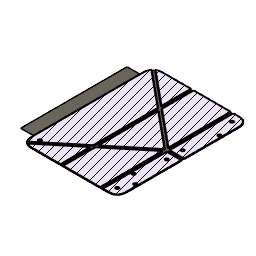
Ipad Case v1 (Autodesk Fusion 360 archive; units mm, degrees)
design "Ipad Cover v2"
part number: 2026-04-06-16-04-37-224
Autodesk Fusion 360 part; units mm, degrees
note: some values were not read from the file. Chosen so that the rebuilt part matches the saved one: which bodies a step acts on. Set by a fixed rule: which sketch regions a step uses.
sketch "Sketch1" plane through (0, 0, 0) normal (0, 0, 1) x (1, 0, 0)
  line L0 (22.75, 0) -> (156.76, 0)
  line L1 (179.51, 22.75) -> (179.51, 223.88)
  line L2 (156.76, 246.63) -> (22.75, 246.63)
  line L3 (0, 223.8801) -> (0, 22.75)
  spline S0 degree 5 poles (22.75, 0) (16.7, 0.14) (14.9, 0.32) (11.36, 0.69) (10.05, 1.08) (8.75, 1.6) (7.46, 2.26) (6.23, 3.06) (5.07, 4) (4.01, 5.05) (3.08, 6.21) (2.27, 7.44) (1.61, 8.73) (1, 10.3) (0.58, 11.86) (0.3, 13.37) (0.14, 14.82) (0.06, 16.18) (0, 22.75) knots 0 0 0 0 0 0 0.071429 0.142857 0.214286 0.285714 0.357143 0.428571 0.5 0.571429 0.642857 0.714286 0.785714 0.857143 0.928571 1 1 1 1 1 1
  line L4 (22.75, 0) -> (16.7, 0.14) construction
  line L5 (16.7, 0.14) -> (14.9, 0.32) construction
  line L6 (14.9, 0.32) -> (11.36, 0.69) construction
  line L7 (11.36, 0.69) -> (10.05, 1.08) construction
  line L8 (10.05, 1.08) -> (8.75, 1.6) construction
  line L9 (8.75, 1.6) -> (7.46, 2.26) construction
  line L10 (7.46, 2.26) -> (6.23, 3.06) construction
  line L11 (6.23, 3.06) -> (5.07, 4) construction
  line L12 (5.07, 4) -> (4.01, 5.05) construction
  line L13 (4.01, 5.05) -> (3.08, 6.21) construction
  line L14 (3.08, 6.21) -> (2.27, 7.44) construction
  line L15 (2.27, 7.44) -> (1.61, 8.73) construction
  line L16 (1.61, 8.73) -> (1, 10.3) construction
  line L17 (1, 10.3) -> (0.58, 11.86) construction
  line L18 (0.58, 11.86) -> (0.3, 13.37) construction
  line L19 (0.3, 13.37) -> (0.14, 14.82) construction
  line L20 (0.14, 14.82) -> (0.06, 16.18) construction
  line L21 (0.06, 16.18) -> (0, 22.75) construction
  spline S1 degree 5 poles (22.75, 0) (16.7, 0.14) (14.9, 0.32) (11.36, 0.69) (10.05, 1.08) (8.75, 1.6) (7.46, 2.26) (6.23, 3.06) (5.07, 4) (4.01, 5.05) (3.08, 6.21) (2.27, 7.44) (1.61, 8.73) (1, 10.3) (0.58, 11.86) (0.3, 13.37) (0.14, 14.82) (0.06, 16.18) (0, 22.75) knots 0 0 0 0 0 0 0.071429 0.142857 0.214286 0.285714 0.357143 0.428571 0.5 0.571429 0.642857 0.714286 0.785714 0.857143 0.928571 1 1 1 1 1 1
  line L22 (22.75, 0) -> (16.7, 0.14) construction
  line L23 (16.7, 0.14) -> (14.9, 0.32) construction
  line L24 (14.9, 0.32) -> (11.36, 0.69) construction
  line L25 (11.36, 0.69) -> (10.05, 1.08) construction
  line L26 (10.05, 1.08) -> (8.75, 1.6) construction
  line L27 (8.75, 1.6) -> (7.46, 2.26) construction
  line L28 (7.46, 2.26) -> (6.23, 3.06) construction
  line L29 (6.23, 3.06) -> (5.07, 4) construction
  line L30 (5.07, 4) -> (4.01, 5.05) construction
  line L31 (4.01, 5.05) -> (3.08, 6.21) construction
  line L32 (3.08, 6.21) -> (2.27, 7.44) construction
  line L33 (2.27, 7.44) -> (1.61, 8.73) construction
  line L34 (1.61, 8.73) -> (1, 10.3) construction
  line L35 (1, 10.3) -> (0.58, 11.86) construction
  line L36 (0.58, 11.86) -> (0.3, 13.37) construction
  line L37 (0.3, 13.37) -> (0.14, 14.82) construction
  line L38 (0.14, 14.82) -> (0.06, 16.18) construction
  line L39 (0.06, 16.18) -> (0, 22.75) construction
  spline S2 degree 5 poles (0, 223.88) (0, 223.8801) (0, 223.8802) (0, 223.8803) (0, 223.8804) (0, 223.8804) knots 0 0 0 0 0 0 0.000083 0.000083 0.000083 0.000083 0.000083 0.000083
  line L40 (0, 223.88) -> (0, 223.88)
  line L41 (0, 223.8804) -> (0, 223.8805)
  line L42 (89.755, 246.63) -> (89.755, 0) construction
  line L43 (179.51, 123.315) -> (0, 123.315) construction
  spline S3 degree 5 poles (156.76, 0) (162.81, 0.14) (164.61, 0.32) (168.15, 0.69) (169.46, 1.08) (170.76, 1.6) (172.05, 2.26) (173.28, 3.06) (174.44, 4) (175.5, 5.05) (176.43, 6.21) (177.24, 7.44) (177.9, 8.73) (178.51, 10.3) (178.93, 11.86) (179.21, 13.37) (179.37, 14.82) (179.45, 16.18) (179.51, 22.75) knots 0 0 0 0 0 0 0.071429 0.142857 0.214286 0.285714 0.357143 0.428571 0.5 0.571429 0.642857 0.714286 0.785714 0.857143 0.928571 1 1 1 1 1 1
  line L44 (156.76, 0) -> (162.81, 0.14) construction
  line L45 (162.81, 0.14) -> (164.61, 0.32) construction
  line L46 (164.61, 0.32) -> (168.15, 0.69) construction
  line L47 (168.15, 0.69) -> (169.46, 1.08) construction
  line L48 (169.46, 1.08) -> (170.76, 1.6) construction
  line L49 (170.76, 1.6) -> (172.05, 2.26) construction
  line L50 (172.05, 2.26) -> (173.28, 3.06) construction
  line L51 (173.28, 3.06) -> (174.44, 4) construction
  line L52 (174.44, 4) -> (175.5, 5.05) construction
  line L53 (175.5, 5.05) -> (176.43, 6.21) construction
  line L54 (176.43, 6.21) -> (177.24, 7.44) construction
  line L55 (177.24, 7.44) -> (177.9, 8.73) construction
  line L56 (177.9, 8.73) -> (178.51, 10.3) construction
  line L57 (178.51, 10.3) -> (178.93, 11.86) construction
  line L58 (178.93, 11.86) -> (179.21, 13.37) construction
  line L59 (179.21, 13.37) -> (179.37, 14.82) construction
  line L60 (179.37, 14.82) -> (179.45, 16.18) construction
  line L61 (179.45, 16.18) -> (179.51, 22.75) construction
  spline S4 degree 5 poles (156.76, 246.63) (162.81, 246.49) (164.61, 246.31) (168.15, 245.94) (169.46, 245.55) (170.76, 245.03) (172.05, 244.37) (173.28, 243.57) (174.44, 242.63) (175.5, 241.58) (176.43, 240.42) (177.24, 239.19) (177.9, 237.9) (178.51, 236.33) (178.93, 234.77) (179.21, 233.26) (179.37, 231.81) (179.45, 230.45) (179.51, 223.88) knots 0 0 0 0 0 0 0.071429 0.142857 0.214286 0.285714 0.357143 0.428571 0.5 0.571429 0.642857 0.714286 0.785714 0.857143 0.928571 1 1 1 1 1 1
  line L62 (156.76, 246.63) -> (162.81, 246.49) construction
  line L63 (162.81, 246.49) -> (164.61, 246.31) construction
  line L64 (164.61, 246.31) -> (168.15, 245.94) construction
  line L65 (168.15, 245.94) -> (169.46, 245.55) construction
  line L66 (169.46, 245.55) -> (170.76, 245.03) construction
  line L67 (170.76, 245.03) -> (172.05, 244.37) construction
  line L68 (172.05, 244.37) -> (173.28, 243.57) construction
  line L69 (173.28, 243.57) -> (174.44, 242.63) construction
  line L70 (174.44, 242.63) -> (175.5, 241.58) construction
  line L71 (175.5, 241.58) -> (176.43, 240.42) construction
  line L72 (176.43, 240.42) -> (177.24, 239.19) construction
  line L73 (177.24, 239.19) -> (177.9, 237.9) construction
  line L74 (177.9, 237.9) -> (178.51, 236.33) construction
  line L75 (178.51, 236.33) -> (178.93, 234.77) construction
  line L76 (178.93, 234.77) -> (179.21, 233.26) construction
  line L77 (179.21, 233.26) -> (179.37, 231.81) construction
  line L78 (179.37, 231.81) -> (179.45, 230.45) construction
  line L79 (179.45, 230.45) -> (179.51, 223.88) construction
  spline S5 degree 5 poles (22.75, 246.63) (16.7, 246.49) (14.9, 246.31) (11.36, 245.94) (10.05, 245.55) (8.75, 245.03) (7.46, 244.37) (6.23, 243.57) (5.07, 242.63) (4.01, 241.58) (3.08, 240.42) (2.27, 239.19) (1.61, 237.9) (1, 236.33) (0.58, 234.77) (0.3, 233.26) (0.14, 231.81) (0.06, 230.45) (0, 223.88) knots 0 0 0 0 0 0 0.071429 0.142857 0.214286 0.285714 0.357143 0.428571 0.5 0.571429 0.642857 0.714286 0.785714 0.857143 0.928571 1 1 1 1 1 1
  line L80 (22.75, 246.63) -> (16.7, 246.49) construction
  line L81 (16.7, 246.49) -> (14.9, 246.31) construction
  line L82 (14.9, 246.31) -> (11.36, 245.94) construction
  line L83 (11.36, 245.94) -> (10.05, 245.55) construction
  line L84 (10.05, 245.55) -> (8.75, 245.03) construction
  line L85 (8.75, 245.03) -> (7.46, 244.37) construction
  line L86 (7.46, 244.37) -> (6.23, 243.57) construction
  line L87 (6.23, 243.57) -> (5.07, 242.63) construction
  line L88 (5.07, 242.63) -> (4.01, 241.58) construction
  line L89 (4.01, 241.58) -> (3.08, 240.42) construction
  line L90 (3.08, 240.42) -> (2.27, 239.19) construction
  line L91 (2.27, 239.19) -> (1.61, 237.9) construction
  line L92 (1.61, 237.9) -> (1, 236.33) construction
  line L93 (1, 236.33) -> (0.58, 234.77) construction
  line L94 (0.58, 234.77) -> (0.3, 233.26) construction
  line L95 (0.3, 233.26) -> (0.14, 231.81) construction
  line L96 (0.14, 231.81) -> (0.06, 230.45) construction
  line L97 (0.06, 230.45) -> (0, 223.88) construction
  dimension "d13" = 22.75
  dimension "d14" = 16.7
  dimension "d15" = 14.9
  dimension "d16" = 11.36
  dimension "d17" = 10.05
  dimension "d18" = 8.75
  dimension "d19" = 7.46
  dimension "d20" = 6.23
  dimension "d21" = 5.07
  dimension "d22" = 4.01
  dimension "d23" = 3.08
  dimension "d24" = 2.27
  dimension "d25" = 1.61
  dimension "d26" = 1
  dimension "d27" = 0.58
  dimension "d28" = 0.3
  dimension "d29" = 0.14
  dimension "d30" = 0.06
  dimension "d31" = 0.14
  dimension "d32" = 0.32
  dimension "d33" = 0.69
  dimension "d34" = 1.08
  dimension "d35" = 1.6
  dimension "d36" = 2.26
  dimension "d37" = 3.06
  dimension "d38" = 4
  dimension "d39" = 5.05
  dimension "d40" = 6.21
  dimension "d41" = 7.44
  dimension "d42" = 8.73
  dimension "d43" = 10.3
  dimension "d44" = 11.86
  dimension "d45" = 13.37
  dimension "d46" = 14.82
  dimension "d47" = 16.18
  dimension "d48" = 22.75
  constraint horizontal L0
  constraint vertical L1
  constraint horizontal L2
  constraint vertical L3
  constraint coincident L3 S2.start
  constraint coincident L3 S2.end
  constraint midpoint S2.start L40
  constraint midpoint S2.end L41
  constraint symmetric L0.start L42 L0.end
  constraint symmetric L3.end L42 L1.start
  constraint symmetric S1 L42 S3
  constraint symmetric L0.start L43 L2.end
  constraint symmetric L3.end L43 S2.start
  constraint symmetric S0 L43 S5
  constraint symmetric L43 L0.end L2.start
  constraint symmetric L43 L1.start L1.end
  constraint symmetric L43 S3 S4
  constraint coincident S2 L3.start
  measures "d13" distance of L3 L0.start
  measures "d14" distance of L3 L4.end
  measures "d15" distance of L3 L5.end
  measures "d16" distance of L3 L6.end
  measures "d17" distance of L3 L7.end
  measures "d18" distance of L3 L8.end
  measures "d19" distance of L3 L9.end
  measures "d20" distance of L3 L10.end
  measures "d21" distance of L3 L11.end
  measures "d22" distance of L3 L12.end
  measures "d23" distance of L3 L13.end
  measures "d24" distance of L3 L14.end
  measures "d25" distance of L3 L15.end
  measures "d26" distance of L3 L16.end
  measures "d27" distance of L3 L17.end
  measures "d28" distance of L3 L18.end
  measures "d29" distance of L3 L19.end
  measures "d30" distance of L3 L20.end
  measures "d31" distance of L0 L4.end
  measures "d32" distance of L0 L5.end
  measures "d33" distance of L0 L6.end
  measures "d34" distance of L0 L7.end
  measures "d35" distance of L0 L8.end
  measures "d36" distance of L0 L9.end
  measures "d37" distance of L0 L10.end
  measures "d38" distance of L0 L11.end
  measures "d39" distance of L0 L12.end
  measures "d40" distance of L0 L13.end
  measures "d41" distance of L0 L14.end
  measures "d42" distance of L0 L15.end
  measures "d43" distance of L0 L16.end
  measures "d44" distance of L0 L17.end
  measures "d45" distance of L0 L18.end
  measures "d46" distance of L0 L19.end
  measures "d47" distance of L0 L20.end
  measures "d48" distance of L0 L3.end
sketch "Sketch2" plane through (0, 0, 0) normal (0, 0, 1) x (1, 0, 0)
  line L0 (22.75, 0) -> (156.76, 0)
  line L1 (179.51, 22.75) -> (179.51, 223.88)
  spline S0 degree 5 poles (156.76, 0) (162.81, 0.14) (164.61, 0.32) (168.15, 0.69) (169.46, 1.08) (170.76, 1.6) (172.05, 2.26) (173.28, 3.06) (174.44, 4) (175.5, 5.05) (176.43, 6.21) (177.24, 7.44) (177.9, 8.73) (178.51, 10.3) (178.93, 11.86) (179.21, 13.37) (179.37, 14.82) (179.45, 16.18) (179.51, 22.75) knots 0 0 0 0 0 0 0.071429 0.142857 0.214286 0.285714 0.357143 0.428571 0.5 0.571429 0.642857 0.714286 0.785714 0.857143 0.928571 1 1 1 1 1 1
  spline S1 degree 5 poles (22.75, 0) (16.7, 0.14) (14.9, 0.32) (11.36, 0.69) (10.05, 1.08) (8.75, 1.6) (7.46, 2.26) (6.23, 3.06) (5.07, 4) (4.01, 5.05) (3.08, 6.21) (2.27, 7.44) (1.61, 8.73) (1, 10.3) (0.58, 11.86) (0.3, 13.37) (0.14, 14.82) (0.06, 16.18) (0, 22.75) knots 0 0 0 0 0 0 0.071429 0.142857 0.214286 0.285714 0.357143 0.428571 0.5 0.571429 0.642857 0.714286 0.785714 0.857143 0.928571 1 1 1 1 1 1
  line L2 (0, 223.8801) -> (0, 22.75)
  line L3 (156.76, 246.63) -> (22.75, 246.63)
  spline S2 degree 5 poles (156.76, 246.63) (162.81, 246.49) (164.61, 246.31) (168.15, 245.94) (169.46, 245.55) (170.76, 245.03) (172.05, 244.37) (173.28, 243.57) (174.44, 242.63) (175.5, 241.58) (176.43, 240.42) (177.24, 239.19) (177.9, 237.9) (178.51, 236.33) (178.93, 234.77) (179.21, 233.26) (179.37, 231.81) (179.45, 230.45) (179.51, 223.88) knots 0 0 0 0 0 0 0.071429 0.142857 0.214286 0.285714 0.357143 0.428571 0.5 0.571429 0.642857 0.714286 0.785714 0.857143 0.928571 1 1 1 1 1 1
  spline S3 degree 5 poles (22.75, 246.63) (16.7, 246.49) (14.9, 246.31) (11.36, 245.94) (10.05, 245.55) (8.75, 245.03) (7.46, 244.37) (6.23, 243.57) (5.07, 242.63) (4.01, 241.58) (3.08, 240.42) (2.27, 239.19) (1.61, 237.9) (1, 236.33) (0.58, 234.77) (0.3, 233.26) (0.14, 231.81) (0.06, 230.45) (0, 223.88) knots 0 0 0 0 0 0 0.071429 0.142857 0.214286 0.285714 0.357143 0.428571 0.5 0.571429 0.642857 0.714286 0.785714 0.857143 0.928571 1 1 1 1 1 1
  line L4 (22.75, 0) -> (156.76, 0) construction
  line L5 (89.755, 246.63) -> (89.755, 0)
  line L6 (179.51, 123.315) -> (0, 123.315)
  line L7 (149.51, 246.63) -> (149.51, 0) construction
  line L8 (74.55, 246.63) -> (74.55, 0) construction
  line L9 (149.51, 123.315) -> (0, 246.63) construction
  line L10 (147.01, 118.0124) -> (147.01, 0)
  line L11 (147.01, 246.63) -> (147.01, 128.6176)
  line L12 (72.05, 56.1858) -> (72.05, 0)
  line L13 (147.01, 118.0124) -> (77.05, 60.3098)
  line L14 (72.05, 56.1858) -> (7.0344, 2.5613)
  line L15 (77.05, 60.3098) -> (77.05, 0)
  line L16 (145.581, 123.315) -> (77.05, 66.791)
  line L17 (72.05, 62.6671) -> (3.305, 5.9666)
  line L18 (147.5455, 121.6947) -> (74.55, 61.4884) construction
  line L19 (72.05, 59.4264) -> (4.9941, 4.1191) construction
  line L20 (147.01, 128.6176) -> (77.05, 186.3202)
  line L21 (72.05, 190.4442) -> (1.5907, 248.5586)
  line L22 (77.05, 246.63) -> (77.05, 186.3202)
  line L23 (77.05, 179.839) -> (77.05, 66.791)
  line L24 (72.05, 246.63) -> (72.05, 190.4442)
  line L25 (72.05, 183.9629) -> (72.05, 62.6671)
  line L26 (145.581, 123.315) -> (77.05, 179.839)
  line L27 (72.05, 183.9629) -> (-1.5907, 244.7014)
  line L28 (179.51, 125.815) -> (152.01, 125.815)
  line L29 (179.51, 120.815) -> (152.01, 120.815)
  line L30 (152.01, 246.63) -> (152.01, 125.815)
  line L31 (152.01, 120.815) -> (152.01, 0)
  dimension "d61" = 30
  dimension "d62" = 74.55
  constraint horizontal L4
  constraint coincident L0.start S1.start
  constraint coincident L3 L7.start
  constraint coincident L4 L7.end
  constraint perpendicular L4 L7
  constraint coincident L3 L8.start
  constraint coincident L0 L8.end
  constraint perpendicular L0 L8
  constraint coincident L6 L16.start
  constraint collinear L12 L25
  constraint collinear L13 L14
  constraint collinear L15 L23
  constraint collinear L16 L17
  constraint coincident L8 L18.end
  constraint collinear L18 L19
  constraint coincident S1 L14.end
  constraint coincident S1 L19.end
  constraint coincident S1 L17.end
  constraint collinear L20 L21
  constraint collinear L22 L23
  constraint collinear L24 L25
  constraint collinear L26 L27
  constraint collinear L30 L31
  measures "d61" distance of L1 L7
  measures "d62" distance of L2 L8
extrude "Extrude1" add sketch "Sketch1" sketch "Sketch2" along normal blind 0.5 of sketch 2 contours L2 S3 L6 L25 L27 | L3 S3 L5 L6 L20 L21 L22 L23 L24 L25 L26 L27 | L0 L1 S0 L29 L31 | L1 L3 S2 L28 L30 makes body 1
extrude "Extrude2" add sketch "Sketch2" along normal blind 3 separate body contours L0 S1 L12 L14 | L0 L5 L13 L15 | S1 L2 L6 L17 L25 | L0 L5 L10 L13 | L2 S3 L6 L25 L27 | L0 L1 S0 L29 L31 | L5 L6 L16 L23 | L5 L6 L16 | L5 L6 L23 L26 | L5 L6 L26 | L3 S3 L21 L24 | L3 L5 L20 L22 | L3 L5 L11 L20 | L1 L3 S2 L28 L30 makes body 2 at (127.925, 183.6963, 0) makes body 3 at (55.6167, 227.9014, 0) makes body 4 at (24.0167, 177.0527, 0) makes body 5 at (104.1287, 107.9667, 0) makes body 6 at (127.925, 62.9337, 0) makes body 7 at (55.6167, 18.7286, 0) makes body 8 at (161.1767, 198.775, 0) makes body 9 at (161.1767, 47.855, 0)
ref_plane "WorkPlane1" through (89.755, 123.315, 1.5) normal (0, 0, 1) x (1, 0, 0)
combine "Combine2" operation add target body 9 tool bodies 6 1 8 2 4 7 3 5
sketch "Sketch3" plane through (0, 0, 1.5) normal (0, 0, 1) x (1, 0, 0)
  line L0 (156.76, 246.63) -> (22.75, 246.63)
  line L1 (22.75, 0) -> (156.76, 0)
  line L2 (179.51, 22.75) -> (179.51, 223.88)
  line L3 (179.51, 123.315) -> (103.6981, 123.315) construction
  line L4 (89.755, 246.63) -> (89.755, 0) construction
  line L5 (179.51, 123.315) -> (0, 123.315) construction
  circle A0 centre (175.095, 197.215) radius 2.5
  circle A1 centre (175.095, 38.245) radius 2.5
  circle A2 centre (164.51, 231.63) radius 2.5
  circle A3 centre (164.51, 15) radius 2.5
  circle A4 centre (156.735, 53.515) radius 2.5
  circle A5 centre (13.525, 19.825) radius 2.5
  circle A6 centre (164.51, 108.315) radius 2.5
  circle A7 centre (164.51, 138.315) radius 2.5
  dimension "d86" = 2.5
  dimension "d96" = 5
  dimension "d97" = 85.34
  dimension "d98" = 73.9
  dimension "d99" = 5
  dimension "d100" = 85.34
  dimension "d101" = 85.07
  dimension "d102" = 5
  dimension "d103" = 15
  dimension "d104" = 15
  dimension "d105" = 5
  dimension "d106" = 15
  dimension "d107" = 15
  dimension "d108" = 5
  dimension "d109" = 66.98
  dimension "d110" = 69.8
  dimension "d111" = 5
  dimension "d112" = 103.49
  dimension "d113" = 76.23
  dimension "d114" = 5
  dimension "d115" = 15
  dimension "d116" = 15
  dimension "d117" = 5
  dimension "d118" = 15
  dimension "d119" = 15
  constraint midpoint L2 L3.start
  constraint perpendicular L2 L3
  measures "d96" diameter of A0
  measures "d97" distance of L4 A0.centre
  measures "d98" distance of L5 A0.centre
  measures "d99" diameter of A1
  measures "d100" distance of L4 A1.centre
  measures "d101" distance of L5 A1.centre
  measures "d102" diameter of A2
  measures "d103" distance of L0 A2.centre
  measures "d104" distance of L2 A2.centre
  measures "d105" diameter of A3
  measures "d106" distance of L1 A3.centre
  measures "d107" distance of L2 A3.centre
  measures "d108" diameter of A4
  measures "d109" distance of L4 A4.centre
  measures "d110" distance of L3 A4.centre
  measures "d111" diameter of A5
  measures "d112" distance of L5 A5.centre
  measures "d113" distance of L4 A5.centre
  measures "d114" diameter of A6
  measures "d115" distance of L3 A6.centre
  measures "d116" distance of L2 A6.centre
  measures "d117" diameter of A7
  measures "d118" distance of L2 A7.centre
  measures "d119" distance of L3 A7.centre
extrude "Extrude3" cut sketch "Sketch3" along normal mid plane 1 bodies 9
sketch "Sketch4" plane through (0, 0, 0) normal (0, 0, 1) x (1, 0, 0)
  line L0 (0, 223.8801) -> (0, 22.75)
  line L1 (0, 123.3151) -> (0, 73.3151) construction
  line L2 (0, 223.8801) -> (0, 22.75)
  line L3 (0, 22.75) -> (-25, 22.75)
  line L4 (-25, 22.75) -> (-25, 223.8801)
  line L5 (-25, 223.8801) -> (0, 223.8801)
  dimension "d85" = 25
  constraint midpoint L0 L1.start
  constraint parallel L0 L1
  constraint perpendicular L2 L3
  constraint parallel L2 L4
  constraint parallel L3 L5
  constraint coincident L0.end L2.end
  constraint parallel L0 L2
  constraint coincident L0.start L2.start
  measures "d85" distance of L0.start L4.end
extrude "Extrude4" add sketch "Sketch4" along normal blind 0.5 separate body makes body 10
